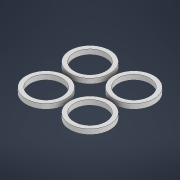
# Autodesk Inventor part: spool_holder_inner_washer
Saved by Autodesk Inventor 2022 (Build 260153000, 153)
## iProperties
Created: 2023-10-01
Part Number: spool_holder_inner_washer
Material: Generic
Document SubType Name: Modeling
Designer: erwin
Density: 1 g/cm^3
Appearance: Default
Author: erwin
Autodesk Inventor part; units mm, degrees
ref_plane "YZ Plane" through (0, 0, 0) normal (1, 0, 0) x (0, 1, 0)
ref_plane "XZ Plane" through (0, 0, 0) normal (0, 1, 0) x (-1, 0, 0)
ref_plane "XY Plane" through (0, 0, 0) normal (0, 0, 1) x (1, 0, 0)
sketch "Sketch1" plane through (0, 0, 0) normal (0, 1, 0) x (-1, 0, 0)
  circle A0 centre (0, 0) radius 4.125
  circle A1 centre (0, 0) radius 3.25
  dimension "d0" = 8.25
  dimension "d1" = 6.5
  constraints: 2 centre point, 2 coincident
  measures "d0" diameter of A0
  measures "d1" diameter of A1
extrude "Extrusion1" add sketch "Sketch1" along normal blind 1
pattern_linear "Rectangular Pattern1" count 2 spacing 9 along (1, 0, 0) count 2 spacing 9 along (0, 0, 1) of "Extrusion1"
body "Solid1"
